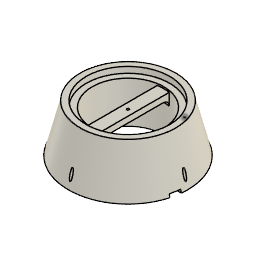
Under Platform (Autodesk Fusion 360 design; units mm, degrees)
Autodesk Fusion 360 part; units mm, degrees
sketch "Sketch1" plane through (0, 0, 0) normal (0, 0, 1) x (1, 0, 0)
  circle A0 centre (0, 0) radius 100
  dimension "d1" = 200
  constraint coincident A0.centre origin
  measures "d1" diameter of A0
ref_plane "WorkPlane1" through (0, 0, 80) normal (0, 0, 1) x (1, 0, 0)
sketch "Sketch2" plane through (0, 0, 80) normal (0, 0, 1) x (1, 0, 0)
  circle A0 centre (0, 0) radius 80
  dimension "d3" = 160
  constraint coincident A0.centre origin
  measures "d3" diameter of A0
loft "Loft1" add profiles "Sketch1", "Sketch2" section 1 section 2 makes body 1
sketch "Sketch3" plane through (0, 0, 80) normal (0, 0, 1) x (-1, 0, 0)
  circle A0 centre (0, 0) radius 80
  circle A1 centre (0, 0) radius 40
  circle A2 centre (0, 0) radius 33.2513
  dimension "d4" = 80
  constraint coincident A0.centre A1.centre
  constraint concentric A1 A2
  measures "d4" diameter of A1
sketch "Sketch4" plane through (0, 0, 0) normal (0, 0, -1) x (1, 0, 0)
  circle A0 centre (0, 0) radius 100
  circle A1 centre (0, 0) radius 65
  dimension "d7" = 130
  constraint coincident A0.centre A1.centre
  measures "d7" diameter of A1
extrude "Extrude2" cut sketch "Sketch3" against normal blind 75 contours A1 bodies 1
sketch "Sketch6" plane through (0, 0, 80) normal (0, 0, 1) x (-1, 0, 0)
  circle A0 centre (0, 0) radius 2.3
  dimension "d10" = 4.6
  constraint coincident A0.centre origin
  measures "d10" diameter of A0
extrude "Extrude3" cut sketch "Sketch6" against normal blind 85 bodies 1
extrude "Extrude4" cut sketch "Sketch4" against normal blind 70 contours A1 bodies 1 makes body 2 at (-22.8104, 1.652, 70)
extrude "Extrude5" cut sketch "Sketch3" against normal blind 10 contours A2 bodies 2
sketch "Sketch8" plane through (0, 0, 80) normal (0, 0, 1) x (-1, 0, 0)
  circle A0 centre (0, 0) radius 80
  circle A1 centre (0, 0) radius 40
  circle A2 centre (0, 0) radius 70
  dimension "d18" = 140
  constraint coincident A0.centre A1.centre
  measures "d18" diameter of A2
extrude "Extrude6" cut sketch "Sketch8" against normal blind 10 contours A2 bodies 1
move_face "OffsetFaces1" offset 5 1 faces at (64.677, 6.4719, 46.6667) on bodies 1
sketch "Sketch9" plane through (0, 0, 0) normal (0, 0, 1) x (1, 0, 0)
  circle A0 centre (0, 95) radius 2.3
  dimension "d22" = 4.6
  measures "d22" diameter of A0
extrude "Extrude7" cut sketch "Sketch9" along normal blind 8 bodies 1
sketch "Sketch11" plane through (0, 0, 8) normal (0, 0, -1) x (1, 0, 0)
  circle A0 centre (0, -95) radius 2.3
  circle A1 centre (0, -95) radius 1
  dimension "d32" = 2
  constraint concentric A0 A1
  measures "d32" diameter of A1
extrude "Extrude9" cut sketch "Sketch11" against normal blind 22 contours A0 | A1 bodies 1
pattern_circular "C-Pattern1" count 4 over 360 about axis through (0, 0, 1.75) along (0, 0, 1) of "Extrude7", "Extrude9"
sketch "Sketch13" plane through (0, 0, 0) normal (0, 1, 0) x (1, 0, 0)
  line L0 (10, -67.1647) -> (-10.1551, -67.1647)
  line L1 (-10.1551, -67.1647) -> (-10.1551, -57.1647)
  line L2 (-10.1551, -57.1647) -> (10, -57.1647)
  line L3 (10, -57.1647) -> (10, -67.1647)
  dimension "d44" = 10
  dimension "d45" = 10
  constraint horizontal L0
  constraint vertical L1
  constraint horizontal L2
  constraint vertical L3
  measures "d44" horizontal distance of origin L2.end
  measures "d45" distance of L0.start L2.end
extrude "Extrude12" add sketch "Sketch13" along normal mid plane 120 bodies 1 2
sketch "Sketch14" plane through (0, 0, 67.1647) normal (0, 0, 1) x (-1, 0, 0)
  arc A0 (10.1551, 59.1344) -> (-10, 59.1608) centre (0, 0) ccw
  line L0 (-10, 59.1608) -> (-10, -59.1608)
  arc A1 (-10, -59.1608) -> (10.1551, -59.1344) centre (0, 0) ccw
  line L1 (10.1551, -59.1344) -> (10.1551, 59.1344)
  circle A2 centre (0, 0) radius 1
  dimension "d48" = 2
  constraint coincident A0.centre A1.centre
  measures "d48" diameter of A2
extrude "Extrude13" cut sketch "Sketch14" against normal blind 17 contours A2 bodies 1
fillet "Fillet2" radius 10 2 edges at (-0.0787, -59.9999, 57.1647) (-0.0787, 59.9999, 57.1647) on bodies 1
sketch "Sketch15" plane through (0, 0, 0) normal (1, 0, 0) x (0, 1, 0)
  line L0 (-9.9291, 0) -> (-25.9291, 0)
  line L1 (-25.9291, 0) -> (-25.9291, 5)
  line L2 (-25.9291, 5) -> (-9.9291, 5)
  line L3 (-9.9291, 5) -> (-9.9291, 0)
  dimension "d55" = 5
  dimension "d56" = 16
  constraint horizontal L0
  constraint vertical L1
  constraint horizontal L2
  constraint vertical L3
  measures "d55" distance of L0.end L1.end
  measures "d56" distance of L0.start L0.end
extrude "Extrude14" cut sketch "Sketch15" along normal blind 126 bodies 1
fillet "Fillet3" radius 1 1 edges at (0.9323, -0.3616, 67.1647) on bodies 1
